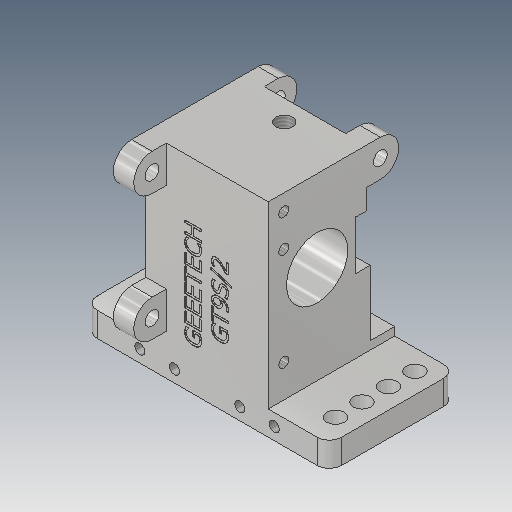
# Autodesk Inventor part: extruder body
Saved by Autodesk Inventor 2019 (Build 230136000, 136)
## iProperties
Created: 2018-11-13
Part Number: extruder body
Material: Aluminum 3004-O
Document SubType Name: Modeling
Designer: LillaHunden
Density: 2.71043 g/cm^3
Appearance: Aluminum - Polished
Mass: 96.6223 g
Surface Area: 137.059 cm^2
Volume: 35.6483 cm^3
Author: LillaHunden
Autodesk Inventor part; units mm, degrees
ref_plane "YZ Plane" through (0, 0, 0) normal (1, 0, 0) x (0, 1, 0)
ref_plane "XZ Plane" through (0, 0, 0) normal (0, 1, 0) x (-1, 0, 0)
ref_plane "XY Plane" through (0, 0, 0) normal (0, 0, 1) x (1, 0, 0)
sketch "Sketch1" plane through (0, 0, 0) normal (0, 0, 1) x (1, 0, 0)
  line L0 (-15, 27.6338) -> (15, 27.6338)
  line L1 (15, 27.6338) -> (15, -16.3662)
  line L2 (-15, -16.3662) -> (-15, 27.6338)
  line L3 (30, -16.3662) -> (30, -22.3662)
  line L4 (30, -22.3662) -> (-30, -22.3662)
  line L5 (-30, -22.3662) -> (-30, -16.3662)
  line L6 (-30, -16.3662) -> (-15, -16.3662)
  line L7 (15, -16.3662) -> (30, -16.3662)
  point P0 (0, 0)
  point P1 (0, -11.858)
  point P2 (0, 27.6338)
  point P3 (0, -11.858)
  dimension "d0" = 60
  dimension "d1" = 6
  dimension "d2" = 30
  dimension "d4" = 50
  dimension "d5" = 15
  constraints: 16 end point, 5 parallel, 3 horizontal, 3 perpendicular, 2 vertical alignment, 1 midpoint
  measures "d0" distance between parallel lines of L3 L5
  measures "d1" distance of L3.start L3.end
  measures "d2" distance of L0.start L0.end
  measures "d4" distance between parallel lines of L4 L0
  measures "d5" distance of L1.end L3.start
extrude "Extrusion1" add sketch "Sketch1" along normal blind 31
sketch "Sketch5" plane through (0, 0, 31) normal (0, 0, 1) x (1, 0, 0)
  line L0 (-5.5191, -14.9346) -> (-5.5191, 16.5611) construction
  line L1 (-5.5191, 16.5611) -> (8.312, 16.5611) construction
  line L2 (8.312, 16.5611) -> (8.312, -14.9346) construction
  line L3 (8.312, -14.9346) -> (-5.5191, -14.9346) construction
  spline S0 degree 2 poles (-1.37, -10.2289) (-1.37, -10.6535) (-1.6293, -11.3569) (-1.8919, -11.6098) knots 0 0 0 1 2 2 2
  spline S1 degree 2 poles (-1.8919, -11.6098) (-2.1577, -11.8626) (-2.9421, -12.1316) (-3.451, -12.1316) knots 0 0 0 1 2 2 2
  spline S2 degree 2 poles (-3.451, -12.1316) (-3.934, -12.1316) (-4.699, -11.8594) (-4.9713, -11.6065) knots 0 0 0 1 2 2 2
  spline S3 degree 2 poles (-4.9713, -11.6065) (-5.2338, -11.3634) (-5.5191, -10.6503) (-5.5191, -10.2257) knots 0 0 0 1 2 2 2
  spline S4 degree 2 poles (-5.5191, -10.2257) (-5.5191, -10.0214) (-5.4607, -9.6519) (-5.4089, -9.4834) knots 0 0 0 1 2 2 2
  spline S5 degree 2 poles (-5.4089, -9.4834) (-5.37, -9.3472) (-5.2274, -9.0166) (-5.1755, -8.9161) knots 0 0 0 1 2 2 2
  line L4 (-5.1755, -8.9161) -> (-4.5337, -8.9161)
  line L5 (-4.5337, -8.9161) -> (-4.5337, -8.9615)
  spline S6 degree 2 poles (-4.5337, -8.9615) (-4.6212, -9.062) (-4.78, -9.2727) (-4.8708, -9.4671) knots 0 0 0 1 2 2 2
  spline S7 degree 2 poles (-4.8708, -9.4671) (-4.9518, -9.6292) (-5.0588, -10.0474) (-5.0588, -10.2872) knots 0 0 0 1 2 2 2
  spline S8 degree 2 poles (-5.0588, -10.2872) (-5.0588, -10.8642) (-4.1901, -11.5774) (-3.4672, -11.5774) knots 0 0 0 1 2 2 2
  spline S9 degree 2 poles (-3.4672, -11.5774) (-3.0653, -11.5774) (-2.4624, -11.3893) (-2.2549, -11.2111) knots 0 0 0 1 2 2 2
  spline S10 degree 2 poles (-2.2549, -11.2111) (-2.0474, -11.0393) (-1.8303, -10.553) (-1.8303, -10.2483) knots 0 0 0 1 2 2 2
  spline S11 degree 2 poles (-1.8303, -10.2483) (-1.8303, -10.0247) (-1.8951, -9.5774) (-1.9599, -9.425) knots 0 0 0 1 2 2 2
  line L6 (-1.9599, -9.425) -> (-2.994, -9.425)
  line L7 (-2.994, -9.425) -> (-2.994, -10.3521)
  line L8 (-2.994, -10.3521) -> (-3.4607, -10.3521)
  line L9 (-3.4607, -10.3521) -> (-3.4607, -8.8999)
  line L10 (-3.4607, -8.8999) -> (-1.7136, -8.8999)
  spline S12 degree 2 poles (-1.7136, -8.8999) (-1.6682, -9.0004) (-1.5288, -9.344) (-1.4867, -9.4898) knots 0 0 0 1 2 2 2
  spline S13 degree 2 poles (-1.4867, -9.4898) (-1.4283, -9.6876) (-1.37, -10.0052) (-1.37, -10.2289) knots 0 0 0 1 2 2 2
  line L11 (-1.4478, -8.2321) -> (-5.4478, -8.2321)
  line L12 (-5.4478, -8.2321) -> (-5.4478, -5.7297)
  line L13 (-5.4478, -5.7297) -> (-4.9745, -5.7297)
  line L14 (-4.9745, -5.7297) -> (-4.9745, -7.7005)
  line L15 (-4.9745, -7.7005) -> (-3.8789, -7.7005)
  line L16 (-3.8789, -7.7005) -> (-3.8789, -5.8626)
  line L17 (-3.8789, -5.8626) -> (-3.4056, -5.8626)
  line L18 (-3.4056, -5.8626) -> (-3.4056, -7.7005)
  line L19 (-3.4056, -7.7005) -> (-1.921, -7.7005)
  line L20 (-1.921, -7.7005) -> (-1.921, -5.7297)
  line L21 (-1.921, -5.7297) -> (-1.4478, -5.7297)
  line L22 (-1.4478, -5.7297) -> (-1.4478, -8.2321)
  line L23 (-1.4478, -5.1462) -> (-5.4478, -5.1462)
  line L24 (-5.4478, -5.1462) -> (-5.4478, -2.6438)
  line L25 (-5.4478, -2.6438) -> (-4.9745, -2.6438)
  line L26 (-4.9745, -2.6438) -> (-4.9745, -4.6146)
  line L27 (-4.9745, -4.6146) -> (-3.8789, -4.6146)
  line L28 (-3.8789, -4.6146) -> (-3.8789, -2.7767)
  line L29 (-3.8789, -2.7767) -> (-3.4056, -2.7767)
  line L30 (-3.4056, -2.7767) -> (-3.4056, -4.6146)
  line L31 (-3.4056, -4.6146) -> (-1.921, -4.6146)
  line L32 (-1.921, -4.6146) -> (-1.921, -2.6438)
  line L33 (-1.921, -2.6438) -> (-1.4478, -2.6438)
  line L34 (-1.4478, -2.6438) -> (-1.4478, -5.1462)
  line L35 (-1.4478, -2.0603) -> (-5.4478, -2.0603)
  line L36 (-5.4478, -2.0603) -> (-5.4478, 0.4421)
  line L37 (-5.4478, 0.4421) -> (-4.9745, 0.4421)
  line L38 (-4.9745, 0.4421) -> (-4.9745, -1.5287)
  line L39 (-4.9745, -1.5287) -> (-3.8789, -1.5287)
  line L40 (-3.8789, -1.5287) -> (-3.8789, 0.3092)
  line L41 (-3.8789, 0.3092) -> (-3.4056, 0.3092)
  line L42 (-3.4056, 0.3092) -> (-3.4056, -1.5287)
  line L43 (-3.4056, -1.5287) -> (-1.921, -1.5287)
  line L44 (-1.921, -1.5287) -> (-1.921, 0.4421)
  line L45 (-1.921, 0.4421) -> (-1.4478, 0.4421)
  line L46 (-1.4478, 0.4421) -> (-1.4478, -2.0603)
  line L47 (-1.4478, 1.9591) -> (-4.9745, 1.9591)
  line L48 (-4.9745, 1.9591) -> (-4.9745, 0.6171)
  line L49 (-4.9745, 0.6171) -> (-5.4478, 0.6171)
  line L50 (-5.4478, 0.6171) -> (-5.4478, 3.8327)
  line L51 (-5.4478, 3.8327) -> (-4.9745, 3.8327)
  line L52 (-4.9745, 3.8327) -> (-4.9745, 2.4907)
  line L53 (-4.9745, 2.4907) -> (-1.4478, 2.4907)
  line L54 (-1.4478, 2.4907) -> (-1.4478, 1.9591)
  line L55 (-1.4478, 4.2379) -> (-5.4478, 4.2379)
  line L56 (-5.4478, 4.2379) -> (-5.4478, 6.7403)
  line L57 (-5.4478, 6.7403) -> (-4.9745, 6.7403)
  line L58 (-4.9745, 6.7403) -> (-4.9745, 4.7695)
  line L59 (-4.9745, 4.7695) -> (-3.8789, 4.7695)
  line L60 (-3.8789, 4.7695) -> (-3.8789, 6.6074)
  line L61 (-3.8789, 6.6074) -> (-3.4056, 6.6074)
  line L62 (-3.4056, 6.6074) -> (-3.4056, 4.7695)
  line L63 (-3.4056, 4.7695) -> (-1.921, 4.7695)
  line L64 (-1.921, 4.7695) -> (-1.921, 6.7403)
  line L65 (-1.921, 6.7403) -> (-1.4478, 6.7403)
  line L66 (-1.4478, 6.7403) -> (-1.4478, 4.2379)
  spline S14 degree 2 poles (-1.3765, 8.8862) (-1.3765, 8.4972) (-1.639, 7.8392) (-1.9016, 7.5993) knots 0 0 0 1 2 2 2
  spline S15 degree 2 poles (-1.9016, 7.5993) (-2.1609, 7.3594) (-2.9389, 7.0969) (-3.4445, 7.0969) knots 0 0 0 1 2 2 2
  spline S16 degree 2 poles (-3.4445, 7.0969) (-3.947, 7.0969) (-4.6925, 7.353) (-4.968, 7.5961) knots 0 0 0 1 2 2 2
  spline S17 degree 2 poles (-4.968, 7.5961) (-5.2371, 7.8359) (-5.5191, 8.4907) (-5.5191, 8.8959) knots 0 0 0 1 2 2 2
  spline S18 degree 2 poles (-5.5191, 8.8959) (-5.5191, 9.0969) (-5.4607, 9.4502) (-5.4154, 9.5993) knots 0 0 0 1 2 2 2
  spline S19 degree 2 poles (-5.4154, 9.5993) (-5.3732, 9.729) (-5.2533, 9.998) (-5.182, 10.1309) knots 0 0 0 1 2 2 2
  line L67 (-5.182, 10.1309) -> (-4.5402, 10.1309)
  line L68 (-4.5402, 10.1309) -> (-4.5402, 10.0888)
  spline S20 degree 2 poles (-4.5402, 10.0888) (-4.605, 10.0175) (-4.7865, 9.797) (-4.874, 9.6382) knots 0 0 0 1 2 2 2
  spline S21 degree 2 poles (-4.874, 9.6382) (-4.9583, 9.4859) (-5.0653, 9.1261) (-5.0653, 8.8927) knots 0 0 0 1 2 2 2
  spline S22 degree 2 poles (-5.0653, 8.8927) (-5.0653, 8.6366) (-4.8546, 8.1795) (-4.6536, 8.0077) knots 0 0 0 1 2 2 2
  spline S23 degree 2 poles (-4.6536, 8.0077) (-4.4494, 7.8392) (-3.8303, 7.6512) (-3.4445, 7.6512) knots 0 0 0 1 2 2 2
  spline S24 degree 2 poles (-3.4445, 7.6512) (-3.0329, 7.6512) (-2.4397, 7.8489) (-2.2355, 8.0207) knots 0 0 0 1 2 2 2
  spline S25 degree 2 poles (-2.2355, 8.0207) (-2.0377, 8.1893) (-1.8368, 8.6398) (-1.8368, 8.8927) knots 0 0 0 1 2 2 2
  spline S26 degree 2 poles (-1.8368, 8.8927) (-1.8368, 9.1228) (-1.9502, 9.515) (-2.0345, 9.6674) knots 0 0 0 1 2 2 2
  spline S27 degree 2 poles (-2.0345, 9.6674) (-2.1188, 9.8132) (-2.2938, 10.0304) (-2.3554, 10.092) knots 0 0 0 1 2 2 2
  line L69 (-2.3554, 10.092) -> (-2.3554, 10.1309)
  line L70 (-2.3554, 10.1309) -> (-1.7201, 10.1309)
  spline S28 degree 2 poles (-1.7201, 10.1309) (-1.6585, 9.998) (-1.545, 9.7646) (-1.4932, 9.5993) knots 0 0 0 1 2 2 2
  spline S29 degree 2 poles (-1.4932, 9.5993) (-1.4348, 9.4243) (-1.3765, 9.1261) (-1.3765, 8.8862) knots 0 0 0 1 2 2 2
  line L71 (-1.4478, 13.5312) -> (-1.4478, 12.9996)
  line L72 (-1.4478, 12.9996) -> (-3.4056, 12.9996)
  line L73 (-3.4056, 12.9996) -> (-3.4056, 11.1585)
  line L74 (-3.4056, 11.1585) -> (-1.4478, 11.1585)
  line L75 (-1.4478, 11.1585) -> (-1.4478, 10.6269)
  line L76 (-1.4478, 10.6269) -> (-5.4478, 10.6269)
  line L77 (-5.4478, 10.6269) -> (-5.4478, 11.1585)
  line L78 (-5.4478, 11.1585) -> (-3.8789, 11.1585)
  line L79 (-3.8789, 11.1585) -> (-3.8789, 12.9996)
  line L80 (-3.8789, 12.9996) -> (-5.4478, 12.9996)
  line L81 (-5.4478, 12.9996) -> (-5.4478, 13.5312)
  line L82 (-5.4478, 13.5312) -> (-1.4478, 13.5312)
  spline S30 degree 2 poles (5.2159, -6.1333) (5.2159, -6.5579) (4.9566, -7.2613) (4.694, -7.5141) knots 0 0 0 1 2 2 2
  spline S31 degree 2 poles (4.694, -7.5141) (4.4282, -7.767) (3.6438, -8.036) (3.1349, -8.036) knots 0 0 0 1 2 2 2
  spline S32 degree 2 poles (3.1349, -8.036) (2.6519, -8.036) (1.8869, -7.7637) (1.6146, -7.5109) knots 0 0 0 1 2 2 2
  spline S33 degree 2 poles (1.6146, -7.5109) (1.3521, -7.2678) (1.0668, -6.5547) (1.0668, -6.13) knots 0 0 0 1 2 2 2
  spline S34 degree 2 poles (1.0668, -6.13) (1.0668, -5.9258) (1.1252, -5.5563) (1.177, -5.3877) knots 0 0 0 1 2 2 2
  spline S35 degree 2 poles (1.177, -5.3877) (1.2159, -5.2516) (1.3585, -4.921) (1.4104, -4.8205) knots 0 0 0 1 2 2 2
  line L83 (1.4104, -4.8205) -> (2.0522, -4.8205)
  line L84 (2.0522, -4.8205) -> (2.0522, -4.8658)
  spline S36 degree 2 poles (2.0522, -4.8658) (1.9647, -4.9663) (1.8059, -5.177) (1.7151, -5.3715) knots 0 0 0 1 2 2 2
  spline S37 degree 2 poles (1.7151, -5.3715) (1.6341, -5.5336) (1.5271, -5.9517) (1.5271, -6.1916) knots 0 0 0 1 2 2 2
  spline S38 degree 2 poles (1.5271, -6.1916) (1.5271, -6.7686) (2.3958, -7.4817) (3.1187, -7.4817) knots 0 0 0 1 2 2 2
  spline S39 degree 2 poles (3.1187, -7.4817) (3.5206, -7.4817) (4.1235, -7.2937) (4.331, -7.1154) knots 0 0 0 1 2 2 2
  spline S40 degree 2 poles (4.331, -7.1154) (4.5384, -6.9436) (4.7556, -6.4574) (4.7556, -6.1527) knots 0 0 0 1 2 2 2
  spline S41 degree 2 poles (4.7556, -6.1527) (4.7556, -5.9291) (4.6908, -5.4817) (4.626, -5.3294) knots 0 0 0 1 2 2 2
  line L85 (4.626, -5.3294) -> (3.5919, -5.3294)
  line L86 (3.5919, -5.3294) -> (3.5919, -6.2564)
  line L87 (3.5919, -6.2564) -> (3.1252, -6.2564)
  line L88 (3.1252, -6.2564) -> (3.1252, -4.8043)
  line L89 (3.1252, -4.8043) -> (4.8723, -4.8043)
  spline S42 degree 2 poles (4.8723, -4.8043) (4.9177, -4.9047) (5.0571, -5.2483) (5.0992, -5.3942) knots 0 0 0 1 2 2 2
  spline S43 degree 2 poles (5.0992, -5.3942) (5.1576, -5.5919) (5.2159, -5.9096) (5.2159, -6.1333) knots 0 0 0 1 2 2 2
  line L90 (5.1381, -3.203) -> (1.6114, -3.203)
  line L91 (1.6114, -3.203) -> (1.6114, -4.5449)
  line L92 (1.6114, -4.5449) -> (1.1381, -4.5449)
  line L93 (1.1381, -4.5449) -> (1.1381, -1.3294)
  line L94 (1.1381, -1.3294) -> (1.6114, -1.3294)
  line L95 (1.6114, -1.3294) -> (1.6114, -2.6714)
  line L96 (1.6114, -2.6714) -> (5.1381, -2.6714)
  line L97 (5.1381, -2.6714) -> (5.1381, -3.203)
  spline S44 degree 2 poles (2.438, -1.1479) (2.13, -1.1479) (1.6179, -0.9469) (1.4331, -0.7718) knots 0 0 0 1 2 2 2
  spline S45 degree 2 poles (1.4331, -0.7718) (1.2548, -0.6065) (1.0571, -0.1235) (1.0571, 0.1228) knots 0 0 0 1 2 2 2
  spline S46 degree 2 poles (1.0571, 0.1228) (1.0571, 0.3983) (1.2418, 0.8457) (1.4169, 1.011) knots 0 0 0 1 2 2 2
  spline S47 degree 2 poles (1.4169, 1.011) (1.6373, 1.2184) (2.3504, 1.4453) (2.8982, 1.4453) knots 0 0 0 1 2 2 2
  spline S48 degree 2 poles (2.8982, 1.4453) (3.3942, 1.4453) (4.2824, 1.2217) (4.5773, 1.0045) knots 0 0 0 1 2 2 2
  spline S49 degree 2 poles (4.5773, 1.0045) (4.8885, 0.7743) (5.2159, 0.1261) (5.2159, -0.3472) knots 0 0 0 1 2 2 2
  spline S50 degree 2 poles (5.2159, -0.3472) (5.2159, -0.4542) (5.1932, -0.6973) (5.1608, -0.801) knots 0 0 0 1 2 2 2
  line L98 (5.1608, -0.801) -> (4.6454, -0.801)
  line L99 (4.6454, -0.801) -> (4.6454, -0.7751)
  spline S51 degree 2 poles (4.6454, -0.7751) (4.6843, -0.707) (4.7524, -0.4218) (4.7524, -0.2759) knots 0 0 0 1 2 2 2
  spline S52 degree 2 poles (4.7524, -0.2759) (4.7524, 0.2492) (4.0587, 0.8489) (3.4169, 0.891) knots 0 0 0 1 2 2 2
  spline S53 degree 2 poles (3.4169, 0.891) (3.5628, 0.6771) (3.6957, 0.2881) (3.6957, 0.058) knots 0 0 0 1 2 2 2
  spline S54 degree 2 poles (3.6957, 0.058) (3.6957, -0.1624) (3.5984, -0.5287) (3.459, -0.7135) knots 0 0 0 1 2 2 2
  spline S55 degree 2 poles (3.459, -0.7135) (3.2937, -0.9274) (2.7913, -1.1479) (2.438, -1.1479) knots 0 0 0 1 2 2 2
  spline S56 degree 2 poles (2.7783, 0.904) (2.3731, 0.904) (1.861, 0.7549) (1.7216, 0.622) knots 0 0 0 1 2 2 2
  spline S57 degree 2 poles (1.7216, 0.622) (1.5919, 0.5053) (1.4947, 0.2622) (1.4947, 0.1196) knots 0 0 0 1 2 2 2
  spline S58 degree 2 poles (1.4947, 0.1196) (1.4947, -0.2111) (1.9679, -0.6033) (2.4153, -0.6033) knots 0 0 0 1 2 2 2
  spline S59 degree 2 poles (2.4153, -0.6033) (2.6681, -0.6033) (2.9955, -0.4736) (3.1122, -0.331) knots 0 0 0 1 2 2 2
  spline S60 degree 2 poles (3.1122, -0.331) (3.1965, -0.2273) (3.2516, 0.0288) (3.2516, 0.1779) knots 0 0 0 1 2 2 2
  spline S61 degree 2 poles (3.2516, 0.1779) (3.2516, 0.3497) (3.1316, 0.7452) (3.0312, 0.8943) knots 0 0 0 1 2 2 2
  spline S62 degree 2 poles (3.0312, 0.8943) (2.9923, 0.8975) (2.8594, 0.904) (2.7783, 0.904) knots 0 0 0 1 2 2 2
  spline S63 degree 2 poles (5.2094, 3.1925) (5.2094, 2.7581) (5.0279, 2.1487) (4.8982, 1.8797) knots 0 0 0 1 2 2 2
  line L100 (4.8982, 1.8797) -> (4.2305, 1.8797)
  line L101 (4.2305, 1.8797) -> (4.2305, 1.9186)
  spline S64 degree 2 poles (4.2305, 1.9186) (4.4769, 2.1812) (4.7491, 2.8457) (4.7491, 3.1536) knots 0 0 0 1 2 2 2
  spline S65 degree 2 poles (4.7491, 3.1536) (4.7491, 3.5944) (4.3829, 4.045) (4.0814, 4.045) knots 0 0 0 1 2 2 2
  spline S66 degree 2 poles (4.0814, 4.045) (3.8415, 4.045) (3.5433, 3.8084) (3.4688, 3.5523) knots 0 0 0 1 2 2 2
  spline S67 degree 2 poles (3.4688, 3.5523) (3.4169, 3.3675) (3.3456, 3.0596) (3.2872, 2.8295) knots 0 0 0 1 2 2 2
  spline S68 degree 2 poles (3.2872, 2.8295) (3.2321, 2.622) (3.0668, 2.2946) (2.9339, 2.1682) knots 0 0 0 1 2 2 2
  spline S69 degree 2 poles (2.9339, 2.1682) (2.801, 2.045) (2.4444, 1.9089) (2.2111, 1.9089) knots 0 0 0 1 2 2 2
  spline S70 degree 2 poles (2.2111, 1.9089) (1.7248, 1.9089) (1.0668, 2.6674) (1.0668, 3.2541) knots 0 0 0 1 2 2 2
  spline S71 degree 2 poles (1.0668, 3.2541) (1.0668, 3.5912) (1.1997, 4.1876) (1.3261, 4.4437) knots 0 0 0 1 2 2 2
  line L102 (1.3261, 4.4437) -> (1.9615, 4.4437)
  line L103 (1.9615, 4.4437) -> (1.9615, 4.4048)
  spline S72 degree 2 poles (1.9615, 4.4048) (1.7864, 4.2136) (1.5271, 3.6171) (1.5271, 3.2897) knots 0 0 0 1 2 2 2
  spline S73 degree 2 poles (1.5271, 3.2897) (1.5271, 2.9202) (1.8739, 2.4632) (2.1559, 2.4632) knots 0 0 0 1 2 2 2
  spline S74 degree 2 poles (2.1559, 2.4632) (2.4088, 2.4632) (2.7102, 2.7322) (2.7783, 2.985) knots 0 0 0 1 2 2 2
  spline S75 degree 2 poles (2.7783, 2.985) (2.8237, 3.1536) (2.9404, 3.6431) (2.989, 3.8051) knots 0 0 0 1 2 2 2
  spline S76 degree 2 poles (2.989, 3.8051) (3.1154, 4.2168) (3.6243, 4.5993) (3.9971, 4.5993) knots 0 0 0 1 2 2 2
  spline S77 degree 2 poles (3.9971, 4.5993) (4.2337, 4.5993) (4.6876, 4.4081) (4.8464, 4.2363) knots 0 0 0 1 2 2 2
  spline S78 degree 2 poles (4.8464, 4.2363) (5.0214, 4.045) (5.2094, 3.5588) (5.2094, 3.1925) knots 0 0 0 1 2 2 2
  line L104 (0.9598, 6.6901) -> (6.0068, 5.1244)
  line L105 (6.0068, 5.1244) -> (6.0068, 4.6706)
  line L106 (6.0068, 4.6706) -> (0.9598, 6.2298)
  line L107 (0.9598, 6.2298) -> (0.9598, 6.6901)
  line L108 (5.1381, 9.5977) -> (5.1381, 7.1309)
  line L109 (5.1381, 7.1309) -> (4.5709, 7.1309)
  spline S79 degree 2 poles (4.5709, 7.1309) (4.3213, 7.3967) (3.8577, 7.87) (3.6081, 8.0969) knots 0 0 0 1 2 2 2
  spline S80 degree 2 poles (3.6081, 8.0969) (3.1057, 8.5539) (2.5028, 8.8878) (2.1819, 8.8878) knots 0 0 0 1 2 2 2
  spline S81 degree 2 poles (2.1819, 8.8878) (2.0133, 8.8878) (1.7605, 8.7841) (1.6794, 8.6901) knots 0 0 0 1 2 2 2
  spline S82 degree 2 poles (1.6794, 8.6901) (1.5984, 8.5961) (1.5174, 8.3497) (1.5174, 8.2006) knots 0 0 0 1 2 2 2
  spline S83 degree 2 poles (1.5174, 8.2006) (1.5174, 8.058) (1.5887, 7.7662) (1.6438, 7.6333) knots 0 0 0 1 2 2 2
  spline S84 degree 2 poles (1.6438, 7.6333) (1.6892, 7.5199) (1.8188, 7.3092) (1.8642, 7.2444) knots 0 0 0 1 2 2 2
  line L110 (1.8642, 7.2444) -> (1.8642, 7.2152)
  line L111 (1.8642, 7.2152) -> (1.2937, 7.2152)
  spline S85 degree 2 poles (1.2937, 7.2152) (1.2127, 7.3805) (1.0538, 7.9737) (1.0538, 8.2395) knots 0 0 0 1 2 2 2
  spline S86 degree 2 poles (1.0538, 8.2395) (1.0538, 8.8003) (1.647, 9.4324) (2.1527, 9.4324) knots 0 0 0 1 2 2 2
  spline S87 degree 2 poles (2.1527, 9.4324) (2.3893, 9.4324) (2.7848, 9.3222) (2.9534, 9.2249) knots 0 0 0 1 2 2 2
  spline S88 degree 2 poles (2.9534, 9.2249) (3.1284, 9.1277) (3.472, 8.8457) (3.6373, 8.6901) knots 0 0 0 1 2 2 2
  spline S89 degree 2 poles (3.6373, 8.6901) (3.9128, 8.4372) (4.5028, 7.8181) (4.6746, 7.6333) knots 0 0 0 1 2 2 2
  line L112 (4.6746, 7.6333) -> (4.6746, 9.5977)
  line L113 (4.6746, 9.5977) -> (5.1381, 9.5977)
  point P0 (0, 0)
  constraints: 2 other
extrude "Extrusion5" cut sketch "Sketch5" against normal blind 0.1
sketch "Sketch6" plane through (0, 0, 0) normal (0, 0, -1) x (-1, 0, 0)
  line L0 (-15, -16.3662) -> (-15, 27.6338) projected
  line L1 (15, 27.6338) -> (15, -16.3662) projected
  line L2 (-15, 27.6338) -> (15, 27.6338)
  line L3 (15, 27.6338) -> (15, -14.3662)
  line L4 (15, -14.3662) -> (-15, -14.3662)
  line L5 (-15, -14.3662) -> (-15, 27.6338)
  line L6 (-30, -22.3662) -> (30, -22.3662) projected
  point P0 (0, 0)
  dimension "d22" = 8
  constraints: 8 end point, 2 parallel, 1 horizontal, 1 perpendicular, 1 point on line
  measures "d22" distance between parallel lines of L6 L4
extrude "Extrusion6" cut sketch "Sketch6" against normal blind 6
sketch "Sketch7" plane through (0, 0, 6) normal (0, 0, -1) x (-1, 0, 0)
  line L0 (0, -5.3662) -> (0, -19.0185) construction
  line L1 (-3, -8.3662) -> (-3, -16.0185)
  line L2 (3, -16.0185) -> (3, -8.3662)
  arc A0 (3, -8.3662) -> (-3, -8.3662) centre (0, -8.3662) ccw
  arc A1 (-3, -16.0185) -> (3, -16.0185) centre (0, -16.0185) ccw
  line L3 (-30, -22.3662) -> (30, -22.3662) projected
  point P0 (0, 0)
  point P1 (0, -12.1924)
  dimension "d25" = 6
  dimension "d26" = 17
  constraints: 8 end point, 7 point on circle, 4 tangent, 2 centre point, 2 point on line, 1 midpoint, 1 parallel, 1 vertical, 1 vertical alignment
  measures "d25" diameter of A1
  measures "d26" distance from line of L3 L0.start
extrude "Extrusion7" add sketch "Sketch7" along normal up to surface (6 mm away)
fillet "Fillet1" radius 2 2 edges at (3, -14.3662, 3) (-3, -14.3662, 3)
sketch "Sketch8" plane through (0, 0, 6) normal (0, 0, -1) x (-1, 0, 0)
  line L0 (-15, 13.6538) -> (15, 13.6538)
  line L1 (15, 13.6538) -> (15, 1.6538)
  line L2 (15, 1.6538) -> (-15, 1.6538)
  line L3 (-15, 1.6538) -> (-15, 13.6538)
  line L4 (-15, 27.6338) -> (15, 27.6338) projected
  line L5 (-15, -14.3662) -> (-15, 27.6338) projected
  line L6 (15, 27.6338) -> (15, -14.3662) projected
  point P0 (0, 0)
  dimension "d30" = 12
  dimension "d31" = 13.98
  constraints: 8 end point, 2 parallel, 2 point on line, 1 horizontal, 1 perpendicular
  measures "d30" distance of L2.end L0.start
  measures "d31" distance between parallel lines of L4 L0
extrude "Extrusion8" cut sketch "Sketch8" against normal blind 3.5 contours L0 L1 L2 L3
sketch "Sketch9" plane through (0, 0, 6) normal (0, 0, -1) x (-1, 0, 0)
  line L0 (-15, 13.6538) -> (15, 13.6538) projected
  line L1 (15, 27.6338) -> (15, 13.6538) projected
  line L2 (-15, 27.6338) -> (15, 27.6338) projected
  line L3 (-15, 13.6538) -> (-15, 27.6338) projected
  point P0 (0, 0)
extrude "Extrusion9" cut sketch "Sketch9" against normal blind 1
sketch "Sketch10" plane through (0, 0, 6) normal (0, 0, -1) x (-1, 0, 0)
  line L0 (-3.5385, 18.6338) -> (3.5385, 18.6338)
  line L1 (3.5385, 18.6338) -> (3.5385, -1.3662)
  line L2 (3.5385, -1.3662) -> (-3.5385, -1.3662)
  line L3 (-3.5385, -1.3662) -> (-3.5385, 18.6338)
  line L4 (-30, -22.3662) -> (30, -22.3662) projected
  line L5 (-15, 27.6338) -> (15, 27.6338) projected
  point P0 (0, 0)
  point P1 (0, 18.6338)
  dimension "d36" = 21
  dimension "d37" = 9
  constraints: 8 end point, 2 parallel, 1 horizontal, 1 midpoint, 1 perpendicular, 1 vertical alignment
  measures "d36" distance between parallel lines of L4 L2
  measures "d37" distance between parallel lines of L5 L0
extrude "Extrusion10" cut sketch "Sketch10" against normal blind 12.5
fillet "Fillet2" radius 1.5 8 edges at (-3.5385, 18.6338, 12.75) (3.5385, 18.6338, 12.75) (0, 18.6338, 18.5) (-3.5385, 8.6338, 18.5) (-3.5385, -1.3662, 12.25) (3.5385, -1.3662, 12.25) (3.5385, 8.6338, 18.5) (0, -1.3662, 18.5)
sketch "Sketch11" plane through (-15, -16.3662, 31) normal (-1, 0, 0) x (0, 0, 1)
  circle A0 centre (-12, 24.02) radius 11.5
  line L0 (-21.5, 30.02) -> (-21.5, 18.02) projected
  line L1 (-24, 44) -> (0, 44) projected
  point P0 (-31, 16.3662)
  point P1 (-21.5, 24.02)
  point P2 (-12, 44)
  dimension "d41" = 23
  constraints: 2 midpoint, 1 centre point, 1 horizontal alignment, 1 vertical alignment
  measures "d41" diameter of A0
extrude "Extrusion11" cut sketch "Sketch11" against normal blind 3.3
sketch "Sketch12" plane through (-11.7, -16.3662, 31) normal (-1, 0, 0) x (0, 0, 1)
  arc A0 (-21.8107, 18.02) -> (-21.8107, 30.02) centre (-12, 24.02) ccw projected
  circle A1 centre (-12, 24.02) radius 7.5
  point P0 (-31, 16.3662)
  dimension "d44" = 15
  constraints: 1 centre point, 1 coincident
  measures "d44" diameter of A1
extrude "Extrusion12" cut sketch "Sketch12" against normal through all
sketch "Sketch13" plane through (-15, -16.3662, 31) normal (-1, 0, 0) x (0, 0, 1)
  line L0 (-32, 39.5) -> (8, 39.5) construction
  line L1 (3.5, 44) -> (-27.5, 44) construction
  arc A0 (-27.5, 44) -> (-27.5, 35) centre (-27.5, 39.5) ccw
  arc A1 (3.5, 35) -> (3.5, 44) centre (3.5, 39.5) ccw
  line L2 (-24, 44) -> (0, 44) construction
  circle A2 centre (-12, 24.02) radius 7.5 construction
  line L3 (-27.5, 35) -> (-24, 35)
  line L4 (-24, 44) -> (-24, 30.02) projected
  line L5 (-14, 35) -> (-24, 35) projected
  line L6 (-24, 30.02) -> (-24, 44) projected
  line L7 (-24, 35) -> (-24, 44)
  line L8 (3.5, 35) -> (0, 35)
  line L9 (0, 0) -> (0, 44) projected
  line L10 (0, 35) -> (0, 44)
  line L11 (-27.5, 44) -> (-24, 44)
  line L12 (0, 44) -> (0, 0) projected
  line L13 (0, 44) -> (3.5, 44)
  point P0 (-31, 16.3662)
  point P1 (-12, 39.5)
  point P2 (-12, 44)
  dimension "d47" = 9
  dimension "d48" = 40
  constraints: 18 end point, 6 point on circle, 4 collinear, 3 horizontal, 3 midpoint, 3 point on line, 2 centre point, 2 tangent, 1 vertical alignment
  measures "d47" diameter of A1
  measures "d48" distance of L0.end L0.start
extrude "Extrusion13" add sketch "Sketch13" against normal blind 5
ref_plane "Work Plane2" through (0, -16.3662, 0) normal (-1, 0, 0) x (0, 0, 1)
mirror "Mirror2" about plane through (0, -16.3662, 0) normal (-1, 0, 0) of "Extrusion13"
sketch "Sketch14" plane through (15, -16.3662, 31) normal (1, 0, 0) x (0, 0, -1)
  circle A0 centre (12, 24.02) radius 7.5 projected
  line L0 (24, 30.02) -> (24, 35) projected
  line L1 (27.5, 35) -> (24, 35) projected
  arc A1 (27.5, 35) -> (27.5, 44) centre (27.5, 39.5) ccw projected
  line L2 (27.5, 44) -> (-3.5, 44) projected
  arc A2 (-3.5, 44) -> (-3.5, 35) centre (-3.5, 39.5) ccw projected
  line L3 (0, 35) -> (-3.5, 35) projected
  line L4 (0, 0) -> (0, 35) projected
  line L5 (31, 0) -> (0, 0) projected
  line L6 (31, 2) -> (31, 0) projected
  line L7 (31, 2) -> (25, 2) projected
  line L8 (25, 2) -> (25, 18.02) projected
  line L9 (25, 18.02) -> (21.5, 18.02) projected
  line L10 (21.5, 18.02) -> (21.5, 30.02) projected
  line L11 (21.5, 30.02) -> (24, 30.02) projected
  line L12 (0, 35) -> (0, 44) projected
  line L13 (0, 35) -> (0, 44)
  point P0 (31, 16.3662)
  constraints: 2 end point, 1 collinear
extrude "Extrusion14" cut sketch "Sketch14" against normal blind 5 contours L12 L3 A2 L2
sketch "Sketch15" plane through (-15, -16.3662, 0) normal (-1, 0, 0) x (0, 0, 1)
  line L0 (18.6319, 8.5) -> (39, 8.5) construction
  line L1 (23.1319, 4) -> (34.5, 4)
  line L2 (34.5, 13) -> (23.1319, 13)
  arc A0 (23.1319, 13) -> (23.1319, 4) centre (23.1319, 8.5) ccw
  arc A1 (34.5, 4) -> (34.5, 13) centre (34.5, 8.5) ccw
  line L3 (31, 35) -> (34.5, 35) projected
  arc A2 (34.5, 35) -> (34.5, 44) centre (34.5, 39.5) ccw projected
  point P0 (0, 16.3662)
  point P1 (28.816, 8.5)
  point P2 (39, 39.5)
  dimension "d53" = 9
  dimension "d54" = 22
  constraints: 8 end point, 8 point on circle, 4 tangent, 2 centre point, 2 point on line, 1 horizontal, 1 midpoint, 1 parallel, 1 vertical alignment
  measures "d53" diameter of A1
  measures "d54" distance between parallel lines of L3 L2
extrude "Extrusion15" add sketch "Sketch15" against normal blind 5
sketch "Sketch16" plane through (-10, 27.6338, 31) normal (0, 1, 0) x (1, 0, 0)
  circle A0 centre (10, 18.925) radius 2.575
  line L0 (14.2529, 21.5) -> (6.6584, 21.5) construction
  line L1 (13.5385, 14) -> (13.5385, 25) projected
  line L2 (20, 24) -> (0, 24) projected
  point P0 (10, 31)
  dimension "d57" = 5.15
  dimension "d58" = 2.5
  constraints: 2 end point, 1 centre point, 1 coincident, 1 perpendicular, 1 tangent, 1 vertical alignment
  measures "d57" diameter of A0
  measures "d58" distance between parallel lines of L2 L0
hole "Hole1" at (0, 27.6338, 12.075) direction (0, -1, 0) diameter 4.134 depth 32 tip angle 118 thread size "M5x0.8" class "6H" standard "ISO Metric profile"
hole "Hole2" at (0, -22.3662, 12.075) direction (0, 1, 0) diameter 4.917 depth 8.7 thread size "M6x1" class "6H" standard "ISO Metric profile"
sketch "Sketch17" plane through (0, -13.6662, 12.075) normal (0, -1, 0) x (1, 0, 0)
  circle A0 centre (0, 0) radius 0.75
  point P0 (0, -12.075)
  dimension "d75" = 1.5
  constraints: 1 centre point
  measures "d75" diameter of A0
extrude "Extrusion16" cut sketch "Sketch17" against normal through all
sketch "Sketch18" plane through (0, 0, 0) normal (0, 0, -1) x (-1, 0, 0)
  arc A0 (3, -8.3662) -> (-3, -8.3662) centre (0, -8.3662) ccw projected
  point P0 (0, 0)
  constraints: 1 coincident
hole "Hole3" at (0, -8.3662, 0) direction (0, 0, 1) diameter 2.459 depth 10 thread size "M3x0.5" class "6H" standard "ISO Metric profile"
sketch "Sketch19" plane through (0, 0, 0) normal (0, 0, -1) x (-1, 0, 0)
  line L0 (0, -16.2637) -> (0, -22.3662) construction
  line L1 (-30, -22.3662) -> (30, -22.3662) projected
  line L2 (-30, -16.3662) -> (-30, -22.3662) projected
  point P0 (0, 0)
  point P1 (-16.5, -19.3662)
  point P2 (-8, -19.3662)
  point P3 (8, -19.3662)
  point P4 (16.5, -19.3662)
  point P5 (-30, -19.3662)
  dimension "d85" = 8.5
  dimension "d86" = 8.5
  dimension "d87" = 13.5
  constraints: 4 horizontal alignment, 2 end point, 2 midpoint, 1 symmetric about line
  measures "d85" distance of point (-8, -19.366) point (-16.5, -19.366)
  measures "d86" distance of point (16.5, -19.366) point (8, -19.366)
  measures "d87" distance from line of L2 point (-16.5, -19.366)
hole "Hole4" at (16.5, -19.3662, 0) at (8, -19.3662, 0) at (-8, -19.3662, 0) at (-16.5, -19.3662, 0) direction (0, 0, 1) diameter 2.459 depth 38.75 thread size "M3x0.5" class "6H" standard "ISO Metric profile"
sketch "Sketch20" plane through (-30, -22.3662, 0) normal (0, -1, 0) x (1, 0, 0)
  line L0 (30, 0) -> (30, 6.5645)
  line L1 (31.2295, 10) -> (31.2295, 0) projected
  line L2 (0, 31) -> (60, 31) projected
  point P0 (5, 5)
  point P1 (55, 5)
  point P2 (55, 11.5)
  point P3 (55, 18)
  point P4 (55, 24.5)
  point P5 (5, 5)
  point P6 (5, 11.5)
  point P7 (5, 18)
  point P8 (5, 24.5)
  dimension "d95" = 50
  dimension "d96" = 6.5
  dimension "d97" = 6.5
  dimension "d98" = 6.5
  dimension "d99" = 6.5
  constraints: 5 symmetric about line, 3 vertical alignment, 2 end point, 1 parallel
  measures "d95" distance of point (55, 5) point (5, 5)
  measures "d96" distance from line of L2 point (55, 24.5)
  measures "d97" distance of point (55, 18) point (55, 24.5)
  measures "d98" distance of point (55, 18) point (55, 11.5)
  measures "d99" distance of point (55, 11.5) point (55, 5)
hole "Hole5" at (-25, -22.3662, 5) at (-25, -22.3662, 24.5) at (-25, -22.3662, 18) at (-25, -22.3662, 11.5) direction (0, 1, 0) diameter 3.242 depth 11.8 thread size "M4x0.7" class "6H" standard "ISO Metric profile"
sketch "Sketch21" plane through (15, -16.3662, 31) normal (1, 0, 0) x (0, 0, -1)
  line L0 (27.5, 44) -> (0, 44) projected
  point P0 (31, 16.3662)
  point P1 (3.7936, 40)
  point P2 (3.7936, 32)
  point P3 (3.7936, 8)
  dimension "d107" = 4
  dimension "d108" = 8
  dimension "d109" = 32
  constraints: 2 vertical alignment
  measures "d107" distance from line of L0 point (3.794, 40)
  measures "d108" distance of point (3.794, 40) point (3.794, 32)
  measures "d109" distance of point (3.794, 40) point (3.794, 8)
hole "Hole6" at (15, 23.6338, 27.2064) at (15, 15.6338, 27.2064) at (15, -8.3662, 27.2064) direction (-1, 0, 0) diameter 2.459 depth 10 thread size "M3x0.5" class "6H" standard "ISO Metric profile"
fillet "Fillet3" radius 3 4 edges at (30, -19.3662, 31) (30, -19.3662, 0) (-30, -19.3662, 0) (-30, -19.3662, 31)
ref_plane "Work Plane3" through (0, -16.3662, 0) normal (-1, 0, 0) x (0, 0, 1)
sketch "Sketch24" plane through (15, -16.3662, 31) normal (1, 0, 0) x (0, 0, -1)
  point P0 (27.5, 39.52)
  point P1 (-3.5, 39.52)
  point P2 (-3.5, 8.52)
hole "Hole8" at (15, 23.1538, 3.5) at (15, 23.1538, 34.5) at (15, -7.8462, 34.5) direction (-1, 0, 0) diameter 3.4 depth 5
sketch "Sketch25" plane through (-15, -16.3662, 0) normal (-1, 0, 0) x (0, 0, 1)
  point P0 (3.5, 39.52)
  point P1 (34.5, 39.52)
  point P2 (34.5, 8.52)
hole "Hole9" at (-15, 23.1538, 3.5) at (-15, 23.1538, 34.5) at (-15, -7.8462, 34.5) direction (1, 0, 0) diameter 3.4 depth 5
sketch "Sketch28" plane through (15, -16.3662, 31) normal (0, 1, 0) x (1, 0, 0)
  circle A0 centre (10, 6.5) radius 2.15
  line L0 (15, 28) -> (15, 3) projected
  line L1 (12, 0) -> (0, 0) projected
  circle A1 centre (10, 13) radius 2.15
  circle A2 centre (10, 19.5) radius 2.15
  circle A3 centre (10, 26) radius 2.15
  point P0 (-15, 31)
  dimension "d157" = 4.3
  dimension "d158" = 5
  dimension "d159" = 6.5
  dimension "d162" = 6.5
  constraints: 4 centre point, 1 vertical, 6 other
  measures "d157" diameter of A0
  measures "d158" distance from line of L0 A0.centre
  measures "d159" distance from line of L1 A0.centre
  measures "d162" distance of A0.centre A1.centre
extrude "Extrusion19" cut sketch "Sketch28" against normal through all
sketch "Sketch29" plane through (-27, -22.3662, 0) normal (0, -1, 0) x (1, 0, 0)
  point P0 (53.8934, -26.0446)
  point P1 (53.8934, -6.0446)
  point P2 (53.8934, 40.0506)
equation "\"d86\" = d85"
equation "\"d97\" = d96"
equation "\"d98\" = d96"
equation "\"d99\" = d96"
body "Solid1"
